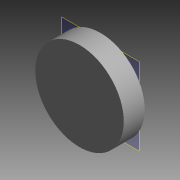
# Autodesk Inventor part: body01
Saved by Autodesk Inventor 2013 (Build 170138000, 138)
## iProperties
Created: 2013-02-19
Part Number: body01
Material: Generic
Document SubType Name: Modeling
Designer: Nano
Density: 1 g/cm^3
Author: Nano
Autodesk Inventor part; units mm, degrees
ref_plane "YZ Plane" through (0, 0, 0) normal (1, 0, 0) x (0, 1, 0)
ref_plane "XZ Plane" through (0, 0, 0) normal (0, 1, 0) x (-1, 0, 0)
ref_plane "XY Plane" through (0, 0, 0) normal (0, 0, 1) x (1, 0, 0)
ref_plane "Work Plane1" through (0, 0, -22.225) normal (0, 0, -1) x (-1, 0, 0)
sketch "Sketch1" plane through (0, 0, -22.225) normal (0, 0, -1) x (-1, 0, 0)
  circle A0 centre (0, 0) radius 147.7423
  line L0 (-195.8977, 76.0742) -> (209.6694, -42.264) construction
  line L1 (-135.6671, 58.4999) -> (-156.0013, 64.4331)
  line L2 (145.8389, -23.6393) -> (172.5523, -31.4338)
  spline S0 degree 4 poles (172.5523, -31.4338) (140.9678, -94.0342) (87.7269, -139.1397) (42.503, -532.8542) (106.3521, -649.2807) (-71.9897, -724.9701) (-159.0807, -904.7553) (-144.6629, -558.7296) (9.1793, -307.9814) (-251.8742, 36.1589) (-156.0013, 64.4331) knots 0 0 0 0 0 0.234794 0.337139 0.431337 0.509169 0.603759 0.711438 1 1 1 1 1
  point P0 (132.692, -105.4544)
  point P1 (82.1143, -291.7082)
  point P2 (74.7064, -566.2438)
  point P3 (60.1104, -648.5122)
  point P4 (-68.3151, -757.5844)
  point P5 (-135.6671, -823.4486)
  point P6 (-145.8342, -757.5844)
  point P7 (-162.8106, -64.6717)
  point P8 (-93.8112, -446.8219)
  constraints: 6 end point, 4 point on line, 2 point on circle, 1 centre point, 1 coincident, 11 other
extrude "Extrusion1" add sketch "Sketch1" against normal blind 69.85 contours A0
body "Solid1"
